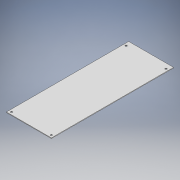
# Autodesk Inventor part: ring_ramp
Saved by Autodesk Inventor 2022 (Build 260153000, 153)
## iProperties
Created: 2021-11-27
Part Number: ring_ramp
Material: Generic
Document SubType Name: Modeling
Designer: carlo
Density: 1 g/cm^3
Appearance: Default
Author: carlo
Autodesk Inventor part; units mm, degrees
ref_plane "YZ Plane" through (0, 0, 0) normal (1, 0, 0) x (0, 1, 0)
ref_plane "XZ Plane" through (0, 0, 0) normal (0, 1, 0) x (-1, 0, 0)
ref_plane "XY Plane" through (0, 0, 0) normal (0, 0, 1) x (1, 0, 0)
sketch "Sketch1" plane through (0, 0, 0) normal (0, 1, 0) x (-1, 0, 0)
  line L0 (0, 0) -> (114.3, 0)
  line L1 (114.3, 0) -> (114.3, -311.15)
  line L2 (114.3, -311.15) -> (0, -311.15)
  line L3 (0, -311.15) -> (0, 0)
  circle A0 centre (107.95, -6.35) radius 2.3114
  circle A1 centre (6.35, -6.35) radius 2.3114
  circle A2 centre (107.95, -298.45) radius 2.3114
  circle A3 centre (6.35, -298.45) radius 2.3114
  dimension "d0" = 114.3
  dimension "d1" = 311.15
  dimension "d2" = 4.6228
  dimension "d3" = 6.35
  dimension "d4" = 6.35
  dimension "d5" = 4.6228
  dimension "d6" = 6.35
  dimension "d7" = 6.35
  dimension "d10" = 4.6228
  dimension "d11" = 6.35
  dimension "d12" = 292.1
  dimension "d13" = 4.6228
  dimension "d14" = 6.35
  dimension "d15" = 0
  constraints: 8 end point, 4 centre point, 2 parallel, 1 horizontal, 1 perpendicular
  measures "d0" distance of L1.end L2.end
  measures "d1" distance of L0.end L1.end
  measures "d2" diameter of A0
  measures "d3" distance from line of L1 A0.centre
  measures "d4" distance from line of A0.centre L0
  measures "d5" diameter of A1
  measures "d6" distance from line of L3 A1.centre
  measures "d7" distance from line of L0 A1.centre
  measures "d10" diameter of A2
  measures "d11" distance from line of L1 A2.centre
  measures "d12" distance of A0.centre A2.centre
  measures "d13" diameter of A3
  measures "d14" distance from line of L3 A3.centre
  measures "d15" vertical distance of A2.centre A3.centre
extrude "Extrusion2" add sketch "Sketch1" along normal blind 1.5875
body "Solid2"
